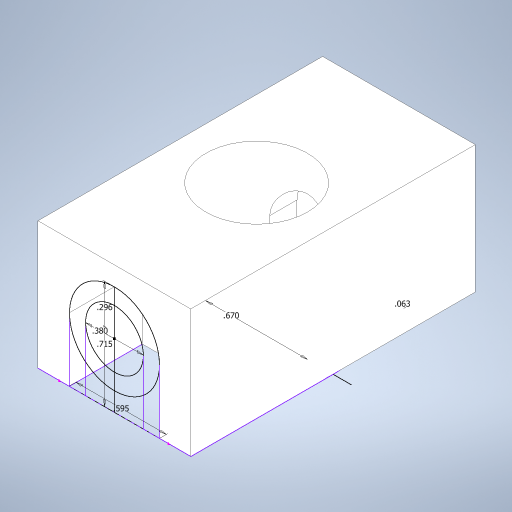
# Autodesk Inventor part: Servo Actuated Ball Valve Shell Torque Test Mount
Saved by Autodesk Inventor 2023 (Build 270158000, 158)
## iProperties
Created: 2023-02-08
Part Number: Servo Actuated Ball Valve Shell Torque Test Mount
Material: Generic
Document SubType Name: Modeling
Designer: tommy
Density: 1 g/cm^3
Appearance: Default
Author: tommy
Autodesk Inventor part; units mm, degrees
ref_plane "YZ Plane" through (0, 0, 0) normal (1, 0, 0) x (0, 1, 0)
ref_plane "XZ Plane" through (0, 0, 0) normal (0, 1, 0) x (-1, 0, 0)
ref_plane "XY Plane" through (0, 0, 0) normal (0, 0, 1) x (1, 0, 0)
sketch "Sketch1" plane through (0, 0, 0) normal (0, 1, 0) x (-1, 0, 0)
  circle A0 centre (0, 0) radius 8.509
  line L0 (7.5565, 23.7871) -> (-7.5565, 23.7871)
  line L1 (7.5565, -23.7871) -> (-7.5565, -23.7871)
  line L2 (7.5565, 23.7871) -> (7.5565, 8.2342)
  line L3 (7.5565, -8.2342) -> (7.5565, -23.7871)
  arc A1 (7.5565, -8.2342) -> (7.5565, 8.2342) centre (0, 0) ccw
  arc A2 (-7.5565, 8.2342) -> (-7.5565, -8.2342) centre (0, 0) ccw
  line L4 (-7.5565, -23.7871) -> (-7.5565, -8.2342)
  line L5 (-7.5565, 8.2342) -> (-7.5565, 23.7871)
  line L6 (-9.144, -8.9047) -> (-9.144, -23.7871)
  line L7 (9.144, -23.7871) -> (9.144, -8.9047)
  arc A3 (9.144, -8.9047) -> (9.144, 8.9047) centre (0, 0) ccw
  line L8 (9.144, 8.9047) -> (9.144, 23.7871)
  line L9 (-9.144, 23.7871) -> (-9.144, 8.9047)
  arc A4 (-9.144, 8.9047) -> (-9.144, -8.9047) centre (0, 0) ccw
  line L10 (7.5565, -23.7871) -> (9.144, -23.7871)
  line L11 (9.144, -23.7871) -> (-9.144, -23.7871)
  line L12 (-7.5565, 23.7871) -> (-9.144, 23.7871)
  line L13 (-9.144, 23.7871) -> (9.144, 23.7871)
  circle A5 centre (0, 0) radius 11.176
  line L14 (16.0553, 0) -> (-15.8373, 0)
  line L15 (12.7635, 0) -> (12.7635, 23.7871)
  line L16 (12.7635, 23.7871) -> (9.144, 23.7871)
  line L17 (-12.7635, 0) -> (-12.7635, 23.7871)
  line L18 (-12.7635, 23.7871) -> (-9.144, 23.7871)
  point P0 (-7.5565, -8.2342)
  point P1 (-7.5565, 8.2342)
  point P2 (-12.7635, 0)
  point P3 (-8.509, 0)
  point P4 (8.509, 0)
  point P5 (12.7635, 0)
  dimension "d0" = 17.018
  dimension "d6" = 15.113
  dimension "d7" = 1.5875
  constraints: 38 end point, 10 point on circle, 7 perpendicular, 6 centre point, 5 point on line, 3 coincident, 3 vertical, 2 horizontal, 2 tangent, 1 concentric
  measures "d0" diameter of A0
  measures "d6" distance of L0.start L0.end
  measures "d7" distance between parallel lines of L4 L6
extrude "Extrusion1" add sketch "Sketch1" along normal blind 18.796 contours A0 L14 A2 A5 A1 | A1 L2 L13 L8 A3 L14 | L14 A4 L9 L12 L5 A2 | A5 L5 L0 L2 picked at (-5.8997, 8.3572)
extrude "Extrusion2" cut sketch "Sketch1" along normal blind 2.286 contours L14 A1 A5 A2 A0 | A0 L14 A2 A5 A1
sketch "Sketch2" plane through (-9.144, 0, 23.7871) normal (0, 0, 1) x (1, 0, 0)
  line L0 (9.144, 0) -> (9.144, 18.161)
  line L1 (9.144, 18.161) -> (9.144, 10.6426)
  circle A0 centre (9.144, 10.6426) radius 7.5184
  line L2 (16.6624, 10.6426) -> (16.6624, 0)
  line L3 (20.32, 0) -> (-2.032, 0) projected
  line L4 (1.6256, 10.6426) -> (1.6256, 0)
  line L5 (1.6256, 0) -> (16.6624, 0)
  circle A1 centre (9.144, 10.6426) radius 4.826
  line L6 (4.318, 10.6426) -> (4.318, 0)
  line L7 (13.97, 10.6426) -> (13.97, 0)
  line L8 (18.288, 0) -> (0, 0) projected
  dimension "d12" = 18.161
  dimension "d13" = 7.5184
  dimension "d17" = 9.652
  constraints: 14 end point, 5 point on circle, 5 point on line, 3 perpendicular, 2 centre point, 2 coincident, 2 vertical, 1 parallel
  measures "d12" distance of L0.start L0.end
  measures "d13" distance of L0.end L1.end
  measures "d17" diameter of A1
extrude "Extrusion3" cut sketch "Sketch2" against normal blind 254 contours L3 L6 A0 L0 | L0 A0 L7 L3 | A0 L6 A1 L0 | L0 A1 L7 A0 | A1 L0 | L0 A1 picked at (8.209, 4.1293) picked at (10.079, 4.1293)
extrude "Extrusion4" cut sketch "Sketch2" against normal blind 12.2174 contours L7 A0 L2 L3 | L3 L4 A0 L6 | A0 L0 A1 L6 | L7 A1 L0 A0 picked at (3.9398, 7.1935) picked at (14.3482, 7.1935)
extrude "Extrusion5" add sketch "Sketch1" along normal blind 18.796 contours A3 L8 L16 L15 | L17 L18 L9 A4
mirror "Mirror2" about plane through (12.7635, 0, 0) normal (0, 0, -1)
sketch "Sketch3" plane through (0, 18.796, 0) normal (0, 1, 0) x (1, 0, 0)
  circle A0 centre (0, 0) radius 8.509
  line L0 (-12.7635, -23.7871) -> (-7.5184, -23.7871) projected
  line L1 (12.7635, -23.7871) -> (12.7635, 23.7871) projected
  line L2 (-12.7635, -23.7871) -> (12.7635, -23.7871)
  line L3 (12.7635, -23.7871) -> (12.7635, 23.7871)
  line L4 (12.7635, 23.7871) -> (-12.7635, 23.7871)
  line L5 (-12.7635, 23.7871) -> (-12.7635, -23.7871)
  constraints: 8 end point, 2 parallel, 1 centre point, 1 coincident, 1 horizontal, 1 perpendicular
extrude "Extrusion6" add sketch "Sketch3" along normal blind 2.54
body "Solid1"
